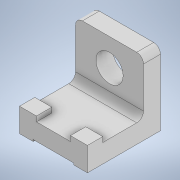
# Autodesk Inventor part: Assignment 2.2 - Tube Mount
Saved by Autodesk Inventor 2021.1 (Build 251245000, 245)
## iProperties
Created: 2021-05-17
Part Number: Assignment 2.2 - Tube Mount
Material: Generic
Document SubType Name: Modeling
Designer: as000166
Density: 1 g/cm^3
Appearance: Default
Author: as000166
Autodesk Inventor part; units mm, degrees
ref_plane "YZ Plane" through (0, 0, 0) normal (1, 0, 0) x (0, 1, 0)
ref_plane "XZ Plane" through (0, 0, 0) normal (0, 1, 0) x (-1, 0, 0)
ref_plane "XY Plane" through (0, 0, 0) normal (0, 0, 1) x (1, 0, 0)
sketch "Sketch1" plane through (0, 0, 0) normal (0, 0, 1) x (1, 0, 0)
  line L0 (0, 0) -> (76.2, 0)
  line L1 (76.2, 0) -> (76.2, -3.175)
  line L2 (76.2, -3.175) -> (101.6, -3.175)
  line L3 (101.6, -3.175) -> (101.6, 41.275)
  line L4 (101.6, 41.275) -> (69.85, 41.275)
  line L5 (69.85, 41.275) -> (69.85, 31.75)
  line L6 (69.85, 31.75) -> (6.35, 31.75)
  line L7 (6.35, 31.75) -> (6.35, 41.275)
  line L8 (6.35, 41.275) -> (-25.4, 41.275)
  line L9 (-25.4, 41.275) -> (-25.4, -3.175)
  line L10 (-25.4, -3.175) -> (0, -3.175)
  line L11 (0, -3.175) -> (0, 0)
  dimension "d0" = 76.2
  dimension "d2" = 25.4
  dimension "d3" = 44.45
  dimension "d4" = 31.75
  dimension "d5" = 9.525
  dimension "d6" = 63.5
  dimension "d8" = 9.525
  dimension "d9" = 31.75
  dimension "d18" = 25.4
  constraints: 24 end point, 7 perpendicular, 2 horizontal, 2 vertical
  measures "d0" distance of L0.start L0.end
  measures "d2" distance of L1.end L2.end
  measures "d3" distance of L2.end L3.end
  measures "d4" distance of L3.end L4.end
  measures "d5" distance of L4.end L5.end
  measures "d6" distance of L5.end L6.end
  measures "d8" distance of L6.end L7.end
  measures "d9" distance of L7.end L8.end
  measures "d18" distance of L9.end L10.end
extrude "Extrusion3" add sketch "Sketch1" against normal blind 136.525
sketch "Sketch5" plane through (101.6, -3.175, 0) normal (1, 0, 0) x (0, 0, -1)
  line L0 (0, 44.45) -> (0, 0) projected
  line L1 (0, 44.45) -> (136.525, 44.45) projected
  line L2 (28.575, 44.45) -> (28.575, 34.925)
  line L3 (136.525, 0) -> (136.525, 44.45) projected
  line L4 (136.525, 44.45) -> (28.575, 44.45)
  line L5 (0, 34.925) -> (136.525, 34.925) projected
  line L6 (28.575, 34.925) -> (136.525, 34.925)
  line L7 (136.525, 34.925) -> (136.525, 44.45)
  point P0 (0, 3.175)
  dimension "d21" = 28.575
  dimension "d22" = 9.525
  constraints: 8 end point, 1 perpendicular, 1 point on line
  measures "d21" distance of L0.start L2.start
  measures "d22" distance of L2.start L2.end
extrude "Extrusion4" cut sketch "Sketch5" against normal through all contours L1 L3 L5 L2
sketch "Sketch6" plane through (101.6, -3.175, 0) normal (1, 0, 0) x (0, 0, -1)
  line L0 (136.525, 0) -> (136.525, 136.525)
  line L1 (136.525, 136.525) -> (104.775, 136.525)
  line L2 (104.775, 136.525) -> (104.775, 0)
  line L3 (0, 0) -> (136.525, 0) projected
  point P0 (0, 3.175)
  dimension "d25" = 136.525
  dimension "d26" = 31.75
  constraints: 6 end point, 2 perpendicular, 1 point on line, 1 vertical
  measures "d25" distance of L0.start L0.end
  measures "d26" distance of L0.end L1.end
extrude "Extrusion5" add sketch "Sketch6" against normal blind 127
sketch "Sketch7" plane through (101.6, -3.175, 0) normal (1, 0, 0) x (0, 0, -1)
  line L0 (28.575, 34.925) -> (28.575, 44.45) projected
  line L1 (28.575, 44.45) -> (28.575, 34.925)
  line L2 (28.575, 34.925) -> (92.075, 34.925)
  line L3 (104.775, 136.525) -> (136.525, 136.525) projected
  line L4 (104.775, 47.625) -> (104.775, 136.525)
  line L5 (104.775, 136.525) -> (136.525, 136.525)
  line L6 (136.525, 136.525) -> (136.525, 0)
  line L7 (136.525, 0) -> (0, 0)
  line L8 (0, 0) -> (0, 44.45)
  line L9 (0, 44.45) -> (28.575, 44.45)
  arc A0 (92.075, 34.925) -> (104.775, 47.625) centre (92.075, 47.625) ccw
  line L10 (28.575, 34.925) -> (28.575, 0)
  line L11 (0, 0) -> (104.775, 0) projected
  point P0 (0, 3.175)
  point P1 (104.775, 34.925)
  point P2 (28.575, 0)
  dimension "d29" = 12.7
  constraints: 18 end point, 6 perpendicular, 3 point on line, 2 collinear, 2 point on circle, 2 tangent, 1 centre point
  measures "d29" radius of A0
extrude "Extrusion6" add sketch "Sketch7" against normal blind 127 contours L2 A0 L4 L3 L6 L7 L10
sketch "Sketch8" plane through (-25.4, 133.35, -104.775) normal (0, 0, 1) x (1, 0, 0)
  line L0 (114.3, 0) -> (12.7, 0)
  line L1 (0, -12.7) -> (0, -88.9)
  line L2 (127, 0) -> (127, -136.525) projected
  arc A0 (127, -12.7) -> (114.3, 0) centre (114.3, -12.7) ccw
  arc A1 (12.7, 0) -> (0, -12.7) centre (12.7, -12.7) ccw
  line L3 (0, -88.9) -> (0, 0) projected
  line L4 (127, 0) -> (0, 0) projected
  line L5 (114.3, 0) -> (127, 0)
  line L6 (127, 0) -> (127, -12.7)
  point P0 (25.4, -133.35)
  point P1 (127, -12.7)
  dimension "d32" = 12.7
  dimension "d33" = 12.7
  constraints: 8 end point, 4 point on circle, 4 tangent, 3 point on line, 2 centre point, 2 collinear, 1 horizontal
  measures "d32" radius of A0
  measures "d33" radius of A1
extrude "Extrusion7" cut sketch "Sketch8" against normal through all contours L4 L2 A0
sketch "Sketch9" plane through (-25.4, 44.45, -104.775) normal (0, 0, 1) x (1, 0, 0)
  line L0 (114.3, 88.9) -> (0, 88.9) projected
  line L1 (12.7, 88.9) -> (69.85, 88.9)
  line L2 (0, 76.2) -> (0, 46.0375)
  line L3 (0, 0) -> (0, 88.9) projected
  arc A0 (12.7, 88.9) -> (0, 76.2) centre (12.7, 76.2) ccw
  line L4 (0, 76.2) -> (0, 88.9)
  point P0 (25.4, -44.45)
  dimension "d36" = 12.7
  constraints: 6 end point, 5 point on line, 3 point on circle, 3 tangent, 1 centre point, 1 collinear
  measures "d36" radius of A0
extrude "Extrusion8" cut sketch "Sketch9" against normal through all
sketch "Sketch10" plane through (-25.4, 44.45, -104.775) normal (0, 0, 1) x (1, 0, 0)
  line L0 (127, 76.2) -> (127, 0) projected
  line L1 (114.3, 88.9) -> (12.7, 88.9) projected
  point P0 (25.4, -44.45)
  point P1 (63.5, 38.1)
  point P2 (63.5, 38.1)
  dimension "d39" = 63.5
  dimension "d40" = 50.8
  constraints: 1 coincident
  measures "d39" distance from line of L0 point (63.5, 38.1)
  measures "d40" distance from line of L1 point (63.5, 38.1)
hole "Hole1" at (38.1, 82.55, -104.775) at (38.1, 82.55, -104.775) direction (0, 0, -1) diameter 50.8 end through all
body "Solid1"
